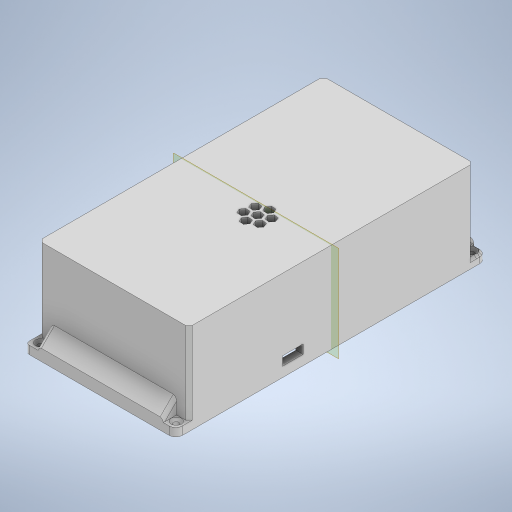
# Autodesk Inventor part: electronics-mount
Saved by Autodesk Inventor 2024 (Build 280153000, 153)
## iProperties
Created: 2024-02-05
Part Number: electronics-mount
Material: Generic
Document SubType Name: Modeling
Designer: crow
Density: 1 g/cm^3
Appearance: Default
Author: crow
## iProperties of the stored document electronics-mount_3DPrint.ipt
Created: 2024-02-08
Part Number: electronics-mount_3DPrint
Material: Generic
Document SubType Name: Modeling
Designer: crow
Density: 1 g/cm^3
Appearance: Default
Author: crow
Autodesk Inventor part; units mm, degrees
ref_plane "YZ Plane" through (0, 0, 0) normal (1, 0, 0) x (0, 1, 0)
ref_plane "XZ Plane" through (0, 0, 0) normal (0, 1, 0) x (-1, 0, 0)
ref_plane "XY Plane" through (0, 0, 0) normal (0, 0, 1) x (1, 0, 0)
sketch "Sketch1" plane through (0, 0, 0) normal (0, 1, 0) x (-1, 0, 0)
  line L0 (-41.6915, 94.55) -> (43.6915, 94.55)
  line L1 (45.6915, 92.55) -> (45.6915, -90.55)
  line L2 (41.6915, -94.55) -> (-41.6915, -94.55)
  line L3 (-45.6915, -90.55) -> (-45.6915, 90.55)
  line L4 (41.305, 89.8895) -> (-41.305, 89.8895) construction
  line L5 (0, 89.8895) -> (0, -90.716948) construction
  line L6 (62.379819, 0) -> (-60.787127, 0) construction
  line L7 (41.305, 89.8895) -> (41.305, -89.8895) construction
  line L8 (41.305, 0) -> (-44.332283, 0) construction
  arc A0 (45.6915, 92.55) -> (43.6915, 94.55) centre (43.6915, 92.55) ccw
  arc A1 (41.6915, -94.55) -> (45.6915, -90.55) centre (41.6915, -90.55) ccw
  arc A2 (-45.6915, -90.55) -> (-41.6915, -94.55) centre (-41.6915, -90.55) ccw
  arc A3 (-41.6915, 94.55) -> (-45.6915, 90.55) centre (-41.6915, 90.55) ccw
  line L9 (41.3045, 84.55) -> (-41.3045, 84.55)
  line L10 (-41.3045, 84.55) -> (-41.3045, -84.55)
  line L11 (-41.3045, -84.55) -> (41.3045, -84.55)
  line L12 (41.3045, -84.55) -> (41.3045, 84.55)
  point P0 (0, 0)
  point P1 (45.6915, -94.55)
  point P2 (45.6915, 94.55)
  point P3 (-45.6915, -94.55)
  point P4 (-41.305, -89.8895)
  dimension "d0" = 91.383
  dimension "d1" = 189.1
  dimension "d2" = 82.61
  dimension "d3" = 179.779
  dimension "d4" = 82.61
  dimension "d5" = 2
  dimension "d6" = 4
  dimension "d16" = 10
  dimension "d17" = 4.387
  dimension "d18" = 10
  dimension "d19" = 4.387
  constraints: 26 end point, 8 point on circle, 8 point on line, 8 tangent, 5 horizontal, 4 centre point, 4 parallel, 2 coincident, 2 equal radius, 2 midpoint, 2 perpendicular, 2 vertical
  measures "d0" distance of point (45.691, -94.55) point (-45.691, -94.55)
  measures "d1" distance of point (45.691, 94.55) point (45.691, -94.55)
  measures "d2" distance of L4.start L4.end
  measures "d3" distance of L4.start L7.end
  measures "d4" distance of point (41.305, -89.889) point (-41.305, -89.889)
  measures "d5" radius of A0
  measures "d6" radius of A1
  measures "d16" distance between parallel lines of L0 L9
  measures "d17" distance between parallel lines of L1 L12
  measures "d18" distance between parallel lines of L2 L11
  measures "d19" distance between parallel lines of L3 L10
extrude "Extrusion1" add sketch "Sketch1" against normal blind 5
hole "Hole1" at (-41.305, 0, 89.8895) at (41.305, 0, 89.8895) at (-41.305, 0, -89.8895) at (41.305, 0, -89.8895) direction (0, -1, 0) diameter 3.4 depth 5 countersink diameter 6.3 countersink angle 90 clearance for "Countersunk Flat Head Screw ISO 2009/7046" size "M3" standard "ISO"
sketch "Sketch2" plane through (0, 0, 0) normal (0, 1, 0) x (1, 0, 0)
  line L0 (-41.3045, -84.55) -> (-41.3045, 84.55)
  line L1 (41.3045, -84.55) -> (-41.3045, -84.55)
  line L2 (41.3045, 84.55) -> (41.3045, -84.55)
  line L3 (-41.3045, 84.55) -> (41.3045, 84.55)
  line L4 (-43.6915, -86.55) -> (43.6915, -86.55)
  line L5 (45.6915, -84.55) -> (45.6915, 84.710496)
  line L6 (43.6915, 86.710496) -> (-43.6915, 86.710496)
  line L7 (-45.6915, 84.710496) -> (-45.6915, -84.55)
  line L8 (-43.6915, -86.55) -> (-45.6915, -84.55)
  line L9 (-45.6915, 84.710496) -> (-43.6915, 86.710496)
  line L10 (45.6915, 84.710496) -> (43.6915, 86.710496)
  line L11 (45.6915, -84.55) -> (43.6915, -86.55)
  line L12 (45.6915, -90.55) -> (45.6915, 90.55)
  line L13 (-45.6915, 90.55) -> (-45.6915, -92.55)
  point P0 (0, 0)
  point P1 (-45.6915, -86.55)
  point P2 (-45.6915, 86.710496)
  point P3 (45.6915, 86.710496)
  point P4 (45.6915, -86.55)
  dimension "d20" = 2
  dimension "d24" = 2
  dimension "d25" = 2
  dimension "d26" = 2
  dimension "d27" = 2
  dimension "d28" = 2
  dimension "d29" = 2
  dimension "d30" = 2
  dimension "d31" = 2
  constraints: 16 end point, 8 point on line, 2 collinear
  measures "d20" distance between parallel lines of L1 L4
  measures "d24" distance of L4.start point (-45.692, -86.55)
  measures "d25" distance of L7.end point (-45.692, -86.55)
  measures "d26" distance of L7.start point (-45.692, 86.71)
  measures "d27" distance of L6.end point (-45.692, 86.71)
  measures "d28" distance of L5.end point (45.691, 86.71)
  measures "d29" distance of L6.start point (45.691, 86.71)
  measures "d30" distance of L5.start point (45.691, -86.55)
  measures "d31" distance of L4.end point (45.691, -86.55)
extrude "Extrusion2" add sketch "Sketch2" along normal blind 40
sketch "Sketch3" plane through (0, 40, 0) normal (0, 1, 0) x (1, 0, 0)
  line L0 (-45.6915, -84.55) -> (-43.6915, -86.55)
  line L1 (-43.6915, -86.55) -> (43.6915, -86.55)
  line L2 (43.6915, -86.55) -> (45.6915, -84.55)
  line L3 (45.6915, -84.55) -> (45.6915, 84.710496)
  line L4 (45.6915, 84.710496) -> (43.6915, 86.710496)
  line L5 (43.6915, 86.710496) -> (-43.6915, 86.710496)
  line L6 (-43.6915, 86.710496) -> (-45.6915, 84.710496)
  line L7 (-45.6915, 84.710496) -> (-45.6915, -84.55)
  line L8 (-41.3045, -84.55) -> (-41.3045, 84.55)
  line L9 (-41.3045, 84.55) -> (41.3045, 84.55)
  line L10 (41.3045, 84.55) -> (41.3045, -84.55)
  line L11 (41.3045, -84.55) -> (-41.3045, -84.55)
  point P0 (0, 0)
extrude "Extrusion3" add sketch "Sketch3" along normal blind 10 contours L7 L6 L5 L4 L3 L2 L1 L0 | L8 L9 L10 L11
sketch "Sketch4" plane through (0, 40, 0) normal (0, -1, 0) x (1, 0, 0)
  circle A0 centre (-16.5, 72.55) radius 2
  line L0 (-41.3045, -84.55) -> (-41.3045, 84.55) projected
  circle A1 centre (16.5, 72.55) radius 2
  circle A2 centre (16.5, -22.45) radius 2
  circle A3 centre (-16, -22.45) radius 2
  line L1 (-24, 74.55) -> (24, 74.55)
  line L2 (24, 74.55) -> (24, -25.45)
  line L3 (24, -25.45) -> (-24, -25.45)
  line L4 (-24, -25.45) -> (-24, 74.55)
  line L5 (-41.3045, 84.55) -> (41.3045, 84.55) projected
  line L6 (16.5, -22.45) -> (-16, -22.45) construction
  line L7 (41.3045, -84.55) -> (-41.3045, -84.55) projected
  line L8 (26.5, -38.55) -> (-26.5, -38.55)
  line L9 (-26.5, -38.55) -> (-26.5, -79.55)
  line L10 (-26.5, -79.55) -> (26.5, -79.55)
  line L11 (26.5, -79.55) -> (26.5, -38.55)
  circle A4 centre (-21.7, -74.75) radius 2
  circle A5 centre (-21.7, -43.35) radius 2
  circle A6 centre (19.7, -67.15) radius 2
  circle A7 centre (19.7, -50.95) radius 2
  point P0 (0, 0)
  point P1 (0, -60.4)
  dimension "d36" = 4
  dimension "d37" = 24.8045
  dimension "d38" = 4
  dimension "d39" = 33
  dimension "d40" = 4
  dimension "d41" = 95
  dimension "d42" = 32.5
  dimension "d43" = 4
  dimension "d44" = 48
  dimension "d45" = 100
  dimension "d46" = 17.3045
  dimension "d47" = 2
  dimension "d48" = 2
  dimension "d49" = 10
  dimension "d54" = 53
  dimension "d55" = 41
  dimension "d56" = 4
  dimension "d57" = 4.8
  dimension "d58" = 4.8
  dimension "d59" = 4
  dimension "d60" = 4.8
  dimension "d61" = 4.8
  dimension "d62" = 4
  dimension "d63" = 6.8
  dimension "d64" = 4
  dimension "d65" = 6.8
  dimension "d66" = 12.4
  dimension "d67" = 12.4
  dimension "d68" = 5
  constraints: 18 end point, 8 centre point, 4 parallel, 3 horizontal, 2 perpendicular
  measures "d36" diameter of A0
  measures "d37" distance from line of L0 A0.centre
  measures "d38" diameter of A1
  measures "d39" distance of A0.centre A1.centre
  measures "d40" diameter of A2
  measures "d41" distance of L6.start A1.centre
  measures "d42" distance of L6.end L6.start
  measures "d43" diameter of A3
  measures "d44" distance of L2.end L3.end
  measures "d45" distance of L1.end L2.end
  measures "d46" distance between parallel lines of L0 L4
  measures "d47" distance from line of L1 A1.centre
  measures "d48" distance from line of L1 A0.centre
  measures "d49" distance between parallel lines of L5 L1
  measures "d54" distance of L10.end L9.end
  measures "d55" distance of L9.end L8.end
  measures "d56" diameter of A4
  measures "d57" distance from line of L10 A4.centre
  measures "d58" distance from line of L9 A4.centre
  measures "d59" diameter of A5
  measures "d60" distance from line of L8 A5.centre
  measures "d61" distance from line of L9 A5.centre
  measures "d62" diameter of A6
  measures "d63" distance from line of L11 A6.centre
  measures "d64" diameter of A7
  measures "d65" distance from line of L11 A7.centre
  measures "d66" distance from line of L10 A6.centre
  measures "d67" distance from line of L8 A7.centre
  measures "d68" distance between parallel lines of L7 L10
extrude "Extrusion4" cut sketch "Sketch4" against normal blind 8.2 contours A0 | A1 | A2 | A3 | A4 | A5 | A6 | A7
sketch "Sketch5" plane through (0, 0, 0) normal (0, 1, 0) x (1, 0, 0)
  line L0 (-41.6915, 94.55) -> (41.6915, 94.55) projected
  line L1 (38.155, 94.55) -> (-38.155, 94.55)
  line L2 (-38.155, 94.55) -> (-38.155, 86.7395)
  line L3 (-38.155, 86.7395) -> (38.155, 86.7395)
  line L4 (38.155, 86.7395) -> (38.155, 94.55)
  circle A0 centre (41.305, 89.8895) radius 3.15 projected
  point P0 (0, 0)
  constraints: 8 end point, 2 parallel, 1 horizontal, 1 perpendicular, 1 point on line, 1 tangent
extrude "Extrusion5" add sketch "Sketch5" along normal blind 10 contours L0 L4 L3 L2
chamfer "Chamfer4" distance 7.81 angle 45 1 edges at (0, 10, -94.55)
chamfer "Chamfer5" distance 1.5 angle 45 6 edges at (-45.6915, 0, -87.6302) (-44.5199, 0, -93.3784) (-39.9232, 0, -94.55) (44.5199, 0, -93.3784) (39.9233, 0, -94.55) (45.6915, 0, -87.6302)
fillet "Fillet1" radius 2 2 edges at (38.155, 6.095, -90.645) (-38.155, 6.095, -90.645)
ref_plane "Work Plane2" through (43.6915, 0, -0.080248) normal (0, 0, -1) x (-1, 0, 0)
mirror "Mirror1" about plane through (43.6915, 0, -0.080248) normal (0, 0, -1) of "Extrusion5", "Fillet1", "Chamfer4"
move faces "Move1" translate (0, 0, 0.160496) faces at (12.051667, 0.73, 94.389504)
sketch "Sketch6" plane through (-45.6915, -5, 92.55) normal (-1, 0, 0) x (0, 0, 1)
  circle A0 centre (-42, 8) radius 6.2
  line L0 (-8, 45) -> (-177.1, 45) projected
  line L1 (-8, 5) -> (-8, 55) projected
  point P0 (-92.55, 5)
  dimension "d96" = 12.4
  dimension "d97" = 37
  dimension "d98" = 34
  constraints: 1 centre point
  measures "d96" diameter of A0
  measures "d97" distance from line of L0 A0.centre
  measures "d98" distance from line of L1 A0.centre
extrude "Extrusion6" cut sketch "Sketch6" against normal blind 10
sketch "Sketch7" plane through (45.6915, -5, 90.55) normal (1, 0, 0) x (0, 0, -1)
  line L0 (61, 6) -> (73.5, 6)
  line L1 (73.5, 6) -> (73.5, 11.5)
  line L2 (73.5, 11.5) -> (61, 11.5)
  line L3 (61, 11.5) -> (61, 6)
  line L4 (175.1, 45) -> (6, 45) projected
  line L5 (181.1, 0) -> (0, 0) projected
  line L6 (6, 5) -> (6, 55) projected
  point P0 (90.55, 5)
  dimension "d101" = 12.5
  dimension "d102" = 5.5
  dimension "d103" = 6
  dimension "d104" = 55
  constraints: 8 end point, 2 parallel, 1 horizontal, 1 perpendicular
  measures "d101" distance of L2.end L1.end
  measures "d102" distance of L1.end L0.end
  measures "d103" distance between parallel lines of L5 L0
  measures "d104" distance between parallel lines of L6 L3
extrude "Extrusion7" cut sketch "Sketch7" against normal blind 10
sketch "Sketch8" plane through (0, 50, 0) normal (0, 1, 0) x (1, 0, 0)
  circle A0 centre (-16.5, -72.55) radius 2
  circle A1 centre (16.5, -72.55) radius 2
  line L0 (-43.6915, -86.55) -> (43.6915, -86.55)
  line L1 (43.6915, -86.55) -> (45.6915, -84.55)
  line L2 (45.6915, -84.55) -> (45.6915, 84.710496)
  line L3 (45.6915, 84.710496) -> (43.6915, 86.710496)
  line L4 (43.6915, 86.710496) -> (-43.6915, 86.710496)
  line L5 (-43.6915, 86.710496) -> (-45.6915, 84.710496)
  line L6 (-45.6915, 84.710496) -> (-45.6915, -84.55)
  line L7 (-45.6915, -84.55) -> (-43.6915, -86.55)
  circle A2 centre (16.5, 22.45) radius 2
  circle A3 centre (-16, 22.45) radius 2
  circle A4 centre (-21.7, 43.35) radius 2
  circle A5 centre (-21.7, 74.75) radius 2
  circle A6 centre (19.7, 67.15) radius 2
  circle A7 centre (19.7, 50.95) radius 2
  line L8 (10.494033, -13.426738) -> (8.264827, -16.442376)
  line L9 (8.264827, -16.442376) -> (4.538604, -16.019647)
  line L10 (4.538604, -16.019647) -> (3.041587, -12.581278)
  line L11 (3.041587, -12.581278) -> (5.270794, -9.565639)
  line L12 (5.270794, -9.565639) -> (8.997017, -9.988369)
  line L13 (8.997017, -9.988369) -> (10.494033, -13.426738)
  line L14 (5.148448, -15.395342) -> (3.887173, -12.797266)
  line L15 (3.887173, -12.797266) -> (5.506535, -10.405931)
  line L16 (5.506535, -10.405931) -> (8.387173, -10.612673)
  line L17 (8.387173, -10.612673) -> (9.648448, -13.21075)
  line L18 (9.648448, -13.21075) -> (8.029085, -15.602084)
  line L19 (8.029085, -15.602084) -> (5.148448, -15.395342)
  line L20 (11.226223, -6.97273) -> (9.729206, -3.534361)
  line L21 (9.729206, -3.534361) -> (6.002983, -3.111631)
  line L22 (6.002983, -3.111631) -> (3.773777, -6.12727)
  line L23 (3.773777, -6.12727) -> (5.270794, -9.565639)
  line L24 (8.997017, -9.988369) -> (11.226223, -6.97273)
  line L25 (6.457478, -3.856682) -> (4.646257, -6.106192)
  line L26 (4.646257, -6.106192) -> (5.688779, -8.79951)
  line L27 (5.688779, -8.79951) -> (8.542522, -9.243318)
  line L28 (8.542522, -9.243318) -> (10.353743, -6.993808)
  line L29 (10.353743, -6.993808) -> (9.311221, -4.30049)
  line L30 (9.311221, -4.30049) -> (6.457478, -3.856682)
  line L31 (5.270794, -9.565639) -> (3.041587, -12.581278)
  line L32 (4.425208, -9.349651) -> (2.805846, -11.740985)
  line L33 (0.283296, -6.544833) -> (3.163933, -6.751575)
  line L34 (2.805846, -11.740985) -> (-0.074792, -11.534243)
  line L35 (3.041587, -12.581278) -> (-0.684636, -12.158548)
  line L36 (0.047554, -5.70454) -> (3.773777, -6.12727)
  line L37 (-0.074792, -11.534243) -> (-1.336067, -8.936167)
  line L38 (-1.336067, -8.936167) -> (0.283296, -6.544833)
  line L39 (-0.684636, -12.158548) -> (-2.181653, -8.720179)
  line L40 (-2.181653, -8.720179) -> (0.047554, -5.70454)
  line L41 (3.163933, -6.751575) -> (4.425208, -9.349651)
  line L42 (4.505967, 0.326738) -> (6.002983, -3.111631)
  line L43 (3.773777, -6.12727) -> (6.002983, -3.111631)
  line L44 (-1.449463, -2.266171) -> (0.047554, -5.70454)
  line L45 (0.46554, -4.938411) -> (3.319283, -5.382219)
  line L46 (-0.576983, -2.245093) -> (0.46554, -4.938411)
  line L47 (3.319283, -5.382219) -> (5.130503, -3.132709)
  line L48 (1.234238, 0.004417) -> (-0.576983, -2.245093)
  line L49 (0.779743, 0.749467) -> (-1.449463, -2.266171)
  line L50 (5.130503, -3.132709) -> (4.087981, -0.439391)
  line L51 (4.087981, -0.439391) -> (1.234238, 0.004417)
  line L52 (4.505967, 0.326738) -> (0.779743, 0.749467)
  line L53 (6.002983, -3.111631) -> (9.729206, -3.534361)
  line L54 (11.958413, -0.518722) -> (9.729206, -3.534361)
  line L55 (6.612827, -2.487327) -> (5.351552, 0.11075)
  line L56 (4.505967, 0.326738) -> (6.735173, 3.342376)
  line L57 (5.351552, 0.11075) -> (6.970915, 2.502084)
  line L58 (11.112827, -0.302734) -> (9.493465, -2.694069)
  line L59 (6.970915, 2.502084) -> (9.851552, 2.295342)
  line L60 (6.735173, 3.342376) -> (10.461396, 2.919647)
  line L61 (9.851552, 2.295342) -> (11.112827, -0.302734)
  line L62 (10.461396, 2.919647) -> (11.958413, -0.518722)
  line L63 (9.493465, -2.694069) -> (6.612827, -2.487327)
  line L64 (9.729206, -3.534361) -> (11.226223, -6.97273)
  line L65 (14.952446, -7.39546) -> (11.226223, -6.97273)
  line L66 (14.952446, -7.39546) -> (17.181653, -4.379821)
  line L67 (17.181653, -4.379821) -> (15.684636, -0.941452)
  line L68 (14.497952, -6.650409) -> (16.309172, -4.400899)
  line L69 (16.309172, -4.400899) -> (15.26665, -1.707581)
  line L70 (11.644209, -6.206601) -> (14.497952, -6.650409)
  line L71 (15.26665, -1.707581) -> (12.412907, -1.263773)
  line L72 (15.684636, -0.941452) -> (11.958413, -0.518722)
  line L73 (10.601686, -3.513283) -> (11.644209, -6.206601)
  line L74 (12.412907, -1.263773) -> (10.601686, -3.513283)
  line L75 (11.226223, -6.97273) -> (9.729206, -3.534361)
  line L76 (10.494033, -13.426738) -> (14.220257, -13.849467)
  line L77 (14.220257, -13.849467) -> (16.449463, -10.833829)
  line L78 (16.449463, -10.833829) -> (14.952446, -7.39546)
  line L79 (14.952446, -7.39546) -> (11.226223, -6.97273)
  line L80 (11.226223, -6.97273) -> (8.997017, -9.988369)
  line L81 (15.576983, -10.854907) -> (14.53446, -8.161589)
  line L82 (14.53446, -8.161589) -> (11.680717, -7.717781)
  line L83 (11.680717, -7.717781) -> (9.869497, -9.967291)
  line L84 (9.869497, -9.967291) -> (10.912019, -12.660609)
  line L85 (10.912019, -12.660609) -> (13.765762, -13.104417)
  line L86 (13.765762, -13.104417) -> (15.576983, -10.854907)
  point P0 (0, 0)
  point P1 (6.76781, -13.004008)
  point P2 (6.76781, -13.004008)
  point P3 (7.5, -6.55)
  point P4 (7.5, -6.55)
  point P5 (1.544571, -9.142909)
  point P6 (1.544571, -9.142909)
  point P7 (2.27676, -2.688901)
  point P8 (2.27676, -2.688901)
  point P9 (8.23219, -0.095992)
  point P10 (8.23219, -0.095992)
  point P11 (13.455429, -3.957091)
  point P12 (13.455429, -3.957091)
  point P13 (12.72324, -10.411099)
  point P14 (12.72324, -10.411099)
  point P15 (-1.433144, -10.439364)
  point P16 (3.790096, -14.300462)
  point P17 (4.51781, -14.096304)
  point P18 (9.01781, -11.911711)
  dimension "d111" = 29
  dimension "d112" = 9
  dimension "d116" = 4.5
  constraints: 158 end point, 66 symmetric about line, 7 coincident, 4 midpoint, 26 other
  measures "d111" vertical distance of A2.centre point (7.5, -6.55)
  measures "d112" horizontal distance of A2.centre point (7.5, -6.55)
  measures "d116" horizontal distance of point (4.518, -14.096) point (9.018, -11.912)
extrude "Extrusion8" cut sketch "Sketch8" against normal blind 10 contours L14 L15 L16 L17 L18 L19 | L30 L29 L28 L27 L26 L25 | L32 L34 L37 L38 L33 L41 | L46 L48 L51 L50 L47 L45 | L55 L57 L59 L61 L58 L63 | L70 L73 L74 L71 L69 L68 | L86 L85 L84 L83 L82 L81
sketch "Sketch9" plane through (43.6915, 0, -86.710496) normal (0, 0, -1) x (-1, 0, 0)
  line L0 (87.383, 0) -> (87.383, 50) construction
  line L1 (0, 0) -> (0, 50) construction
  line L2 (56.6915, 15.57735) -> (54.1915, 14.133975)
  line L3 (54.1915, 14.133975) -> (51.6915, 15.57735)
  line L4 (51.6915, 15.57735) -> (51.6915, 18.464102)
  line L5 (51.6915, 18.464102) -> (54.1915, 19.907477)
  line L6 (54.1915, 19.907477) -> (56.6915, 18.464102)
  line L7 (56.6915, 18.464102) -> (56.6915, 15.57735)
  line L8 (57.6915, 15) -> (54.1915, 12.979274)
  line L9 (54.1915, 12.979274) -> (50.6915, 15)
  line L10 (50.6915, 15) -> (50.6915, 19.041452)
  line L11 (50.6915, 19.041452) -> (54.1915, 21.062178)
  line L12 (54.1915, 21.062178) -> (57.6915, 19.041452)
  line L13 (57.6915, 19.041452) -> (57.6915, 15)
  line L14 (44.6915, 15.57735) -> (47.1915, 14.133975)
  line L15 (47.1915, 14.133975) -> (49.6915, 15.57735)
  line L16 (49.6915, 15.57735) -> (49.6915, 18.464102)
  line L17 (49.6915, 18.464102) -> (47.1915, 19.907477)
  line L18 (47.1915, 19.907477) -> (44.6915, 18.464102)
  line L19 (44.6915, 18.464102) -> (44.6915, 15.57735)
  line L20 (43.6915, 15) -> (47.1915, 12.979274)
  line L21 (47.1915, 12.979274) -> (50.6915, 15)
  line L22 (50.6915, 19.041452) -> (47.1915, 21.062178)
  line L23 (47.1915, 21.062178) -> (43.6915, 19.041452)
  line L24 (43.6915, 19.041452) -> (43.6915, 15)
  line L25 (36.6915, 15) -> (36.6915, 19.041452)
  line L26 (40.1915, 19.907477) -> (42.6915, 18.464102)
  line L27 (42.6915, 18.464102) -> (42.6915, 15.57735)
  line L28 (43.6915, 15) -> (40.1915, 12.979274)
  line L29 (40.1915, 21.062178) -> (43.6915, 19.041452)
  line L30 (42.6915, 15.57735) -> (40.1915, 14.133975)
  line L31 (37.6915, 18.464102) -> (40.1915, 19.907477)
  line L32 (40.1915, 14.133975) -> (37.6915, 15.57735)
  line L33 (37.6915, 15.57735) -> (37.6915, 18.464102)
  line L34 (40.1915, 12.979274) -> (36.6915, 15)
  line L35 (36.6915, 19.041452) -> (40.1915, 21.062178)
  line L36 (29.6915, 19.041452) -> (29.6915, 15)
  line L37 (35.6915, 15.57735) -> (35.6915, 18.464102)
  line L38 (36.6915, 19.041452) -> (33.1915, 21.062178)
  line L39 (33.1915, 12.979274) -> (36.6915, 15)
  line L40 (33.1915, 14.133975) -> (35.6915, 15.57735)
  line L41 (35.6915, 18.464102) -> (33.1915, 19.907477)
  line L42 (33.1915, 19.907477) -> (30.6915, 18.464102)
  line L43 (33.1915, 21.062178) -> (29.6915, 19.041452)
  line L44 (30.6915, 15.57735) -> (33.1915, 14.133975)
  line L45 (29.6915, 15) -> (33.1915, 12.979274)
  line L46 (30.6915, 18.464102) -> (30.6915, 15.57735)
  line L47 (50.6915, 25.969655) -> (48.1915, 24.526279)
  line L48 (48.1915, 24.526279) -> (48.1915, 21.639528)
  line L49 (48.1915, 21.639528) -> (50.6915, 20.196152)
  line L50 (50.6915, 20.196152) -> (53.1915, 21.639528)
  line L51 (53.1915, 21.639528) -> (53.1915, 24.526279)
  line L52 (53.1915, 24.526279) -> (50.6915, 25.969655)
  line L53 (50.6915, 27.124356) -> (47.1915, 25.10363)
  line L54 (47.1915, 25.10363) -> (47.1915, 21.062178)
  line L55 (47.1915, 21.062178) -> (50.6915, 19.041452)
  line L56 (54.1915, 21.062178) -> (54.1915, 25.10363)
  line L57 (54.1915, 25.10363) -> (50.6915, 27.124356)
  line L58 (43.6915, 19.041452) -> (40.1915, 21.062178)
  line L59 (43.6915, 19.041452) -> (47.1915, 21.062178)
  line L60 (43.6915, 25.969655) -> (46.1915, 24.526279)
  line L61 (46.1915, 24.526279) -> (46.1915, 21.639528)
  line L62 (46.1915, 21.639528) -> (43.6915, 20.196152)
  line L63 (43.6915, 20.196152) -> (41.1915, 21.639528)
  line L64 (41.1915, 21.639528) -> (41.1915, 24.526279)
  line L65 (41.1915, 24.526279) -> (43.6915, 25.969655)
  line L66 (40.1915, 21.062178) -> (40.1915, 25.10363)
  line L67 (40.1915, 25.10363) -> (43.6915, 27.124356)
  line L68 (43.6915, 27.124356) -> (47.1915, 25.10363)
  line L69 (33.1915, 21.062178) -> (36.6915, 19.041452)
  line L70 (40.1915, 21.062178) -> (36.6915, 19.041452)
  line L71 (33.1915, 25.10363) -> (33.1915, 21.062178)
  line L72 (34.1915, 24.526279) -> (34.1915, 21.639528)
  line L73 (36.6915, 25.969655) -> (34.1915, 24.526279)
  line L74 (36.6915, 27.124356) -> (33.1915, 25.10363)
  line L75 (39.1915, 21.639528) -> (39.1915, 24.526279)
  line L76 (39.1915, 24.526279) -> (36.6915, 25.969655)
  line L77 (40.1915, 25.10363) -> (36.6915, 27.124356)
  line L78 (36.6915, 20.196152) -> (39.1915, 21.639528)
  line L79 (34.1915, 21.639528) -> (36.6915, 20.196152)
  line L80 (87.383, 50) -> (0, 50) construction
  line L81 (43.6915, 50) -> (43.6915, 10) construction
  line L82 (79.8465, 10) -> (7.5365, 10) construction
  point P0 (43.6915, 0)
  point P1 (54.1915, 17.020726)
  point P2 (56.6915, 17.020726)
  point P3 (54.1915, 17.020726)
  point P4 (57.6915, 17.020726)
  point P5 (47.1915, 17.020726)
  point P6 (44.6915, 17.020726)
  point P7 (47.1915, 17.020726)
  point P8 (43.6915, 17.020726)
  point P9 (40.1915, 17.020726)
  point P10 (40.1915, 17.020726)
  point P11 (42.6915, 17.020726)
  point P12 (33.1915, 17.020726)
  point P13 (33.1915, 17.020726)
  point P14 (30.6915, 17.020726)
  point P15 (50.6915, 23.082904)
  point P16 (51.9415, 25.247967)
  point P17 (50.6915, 23.082904)
  point P18 (52.4415, 26.113993)
  point P19 (43.6915, 23.082904)
  point P20 (42.4415, 25.247967)
  point P21 (43.6915, 23.082904)
  point P22 (41.9415, 26.113993)
  point P23 (36.6915, 23.082904)
  point P24 (36.6915, 23.082904)
  point P25 (37.9415, 25.247967)
  point P26 (38.4415, 26.113993)
  dimension "d117" = 5
  dimension "d118" = 1
  dimension "d120" = 5
  constraints: 158 end point, 77 symmetric about line, 7 coincident, 4 midpoint, 1 collinear, 26 other
  measures "d117" distance between parallel lines of L4 L7
  measures "d118" distance between parallel lines of L13 L7
  measures "d120" distance from line of L82 L20.start
extrude "Extrusion9" cut sketch "Sketch9" against normal blind 10 contours L2 L3 L4 L5 L6 L7 | L19 L18 L17 L16 L15 L14 | L26 L27 L30 L32 L33 L31 | L40 L44 L46 L42 L41 L37 | L52 L51 L50 L49 L48 L47 | L60 L61 L62 L63 L64 L65 | L73 L76 L75 L78 L79 L72
equation "\"d4\" = d2"
equation "\"d17\" = d19"
equation "\"d25\" = d24"
equation "\"d26\" = d24"
equation "\"d27\" = d26"
equation "\"d28\" = d24"
equation "\"d29\" = d28"
equation "\"d30\" = d24"
equation "\"d31\" = d30"
equation "\"d38\" = d36"
equation "\"d40\" = d36"
equation "\"d43\" = d36"
equation "\"d48\" = d47"
body "Solid1"
